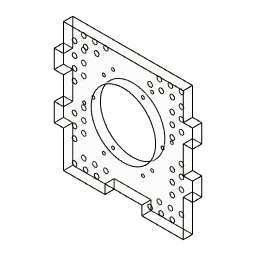
front_and_back_plates (Autodesk Fusion 360 design; units mm, degrees)
Autodesk Fusion 360 part; units mm, degrees
note: some values were not read from the file. Set by a fixed rule: which sketch regions a step uses.
sketch "Esquisse1" plane through (0, 0, 0) normal (0, 1, 0) x (1, 0, 0)
  line L0 (75, 75) -> (-75, 75) construction
  line L1 (-75, 75) -> (-75, -75) construction
  line L2 (-75, -75) -> (75, -75) construction
  line L3 (75, -75) -> (75, 75) construction
  line L4 (75, 75) -> (-75, -75) construction
  line L5 (-75, 75) -> (75, -75) construction
  circle A0 centre (0, 0) radius 35
  circle A1 centre (0, 0) radius 42.5 construction
  circle A2 centre (42.5, 0) radius 1.6
  line L6 (42.5, 0) -> (21.25, 36.8061) construction
  line L7 (21.25, 36.8061) -> (-21.25, 36.8061) construction
  line L8 (-21.25, 36.8061) -> (-42.5, 0) construction
  line L9 (-42.5, 0) -> (-21.25, -36.8061) construction
  line L10 (-21.25, -36.8061) -> (21.25, -36.8061) construction
  line L11 (21.25, -36.8061) -> (42.5, 0) construction
  circle A3 centre (21.25, -36.8061) radius 1.6
  circle A4 centre (-21.25, -36.8061) radius 1.6
  circle A5 centre (-42.5, 0) radius 1.6
  circle A6 centre (-21.25, 36.8061) radius 1.6
  circle A7 centre (21.25, 36.8061) radius 1.6
  line L12 (-65, -65) -> (0, -65)
  line L13 (0, -75) -> (0, 75)
  line L14 (-75, 0) -> (75, 0)
  line L15 (65, -65) -> (0, -65)
  line L16 (-65, 65) -> (0, 65) construction
  line L17 (65, 65) -> (0, 65) construction
  line L18 (-65, 35) -> (-65, 65)
  line L19 (-65, 35) -> (-75, 35)
  line L20 (-75, -75) -> (-75, 75) construction
  line L21 (-75, 15) -> (-65, 15)
  line L22 (-65, 15) -> (-65, 0.2731)
  line L23 (75, 75) -> (75, -75) construction
  line L24 (-75, 15) -> (-75, 35)
  line L25 (-65, -65) -> (-65, -35)
  line L26 (-65, -35) -> (-75, -35)
  line L27 (-75, -15) -> (-65, -15)
  line L28 (-65, -15) -> (-65, 0.2731)
  line L29 (-65, -65) -> (-65, 75) construction
  line L30 (-75, -15) -> (-75, -35)
  line L31 (65, -15) -> (65, 0.2731)
  line L32 (65, -65) -> (65, -35)
  line L33 (75, 15) -> (75, 35)
  line L34 (65, 35) -> (75, 35)
  line L35 (75, -15) -> (75, -35)
  line L36 (75, 15) -> (65, 15)
  line L37 (65, 15) -> (65, 0.2731)
  line L38 (65, -35) -> (75, -35)
  line L39 (65, 35) -> (65, 65)
  line L40 (75, -15) -> (65, -15)
  line L41 (-65, 65) -> (-65, 75)
  line L42 (-65, 75) -> (-20, 75)
  line L43 (-20, 75) -> (-20, 65)
  line L44 (-20, 65) -> (20, 65)
  line L45 (20, 65) -> (20, 75)
  line L46 (20, 75) -> (65, 75)
  line L47 (65, 75) -> (65, 65)
  circle A8 centre (0, 0) radius 50 construction
  point P0 (75, 0)
  point P1 (-75, -25)
  point P2 (-75, 25)
  dimension "d1" = 150
  dimension "d2" = 150
  dimension "d3" = 70
  dimension "d4" = 7.5
  dimension "d5" = 3.2
  dimension "d9" = 10
  dimension "d22" = 20
  dimension "d24" = 20
  dimension "d25" = 10
  dimension "d32" = 40
  dimension "d56" = 15
  dimension "d58" = 50
  constraint horizontal L0
  constraint perpendicular L0 L1
  constraint parallel L1 L3
  constraint coincident L4 A0.centre
  constraint coincident L5 A0.centre
  constraint coincident A0.centre A1.centre
  constraint concentric A0 A1
  constraint coincident A1 A2.centre
  constraint coincident A2.centre L6.start
  constraint coincident L10.end L11.start
  constraint coincident L9.end L10.start
  constraint coincident L8.end L9.start
  constraint coincident L7.end L8.start
  constraint coincident L6.end L7.start
  constraint equal A3 A4
  constraint equal A4 A5
  constraint equal A5 A6
  constraint equal A6 A7
  constraint equal A2 A7
  constraint perpendicular L1 L12
  constraint midpoint L2 L13.start
  constraint midpoint L0 L13.end
  constraint midpoint L1 L14.start
  constraint midpoint L3 P0
  constraint symmetric L12.start L13 L15.start
  constraint symmetric L12.end L13 L15.end
  constraint symmetric L0.start L14 L2.end
  constraint symmetric L0.end L14 L1.end
  constraint symmetric L1.end L14 L0.end
  constraint symmetric L2.end L14 L0.start
  constraint symmetric L12.start L14 L16.start
  constraint symmetric L12.end L14 L16.end
  constraint symmetric L14 L15.start L17.start
  constraint symmetric L14 L12.end L16.end
  constraint coincident A2.centre L14
  constraint perpendicular L12 L25
  constraint coincident L1 L26.end
  constraint perpendicular L1 L26
  constraint coincident L1 L27.start
  constraint perpendicular L1 L27
  constraint perpendicular L14 L28
  constraint coincident L0 L29.end
  constraint perpendicular L0 L29
  constraint coincident L12.start L28
  constraint vertical L24
  constraint coincident L1 L21.start
  constraint symmetric L13 L14.start P0
  constraint symmetric L13 L16.start L17.start
  constraint symmetric L13 L18.start L34.start
  constraint symmetric L13 L19.end L33.end
  constraint symmetric L13 L21.start L33.start
  constraint symmetric L13 L21.end L36.end
  constraint symmetric L13 L22.end L31.end
  constraint symmetric L13 L25.end L32.end
  constraint symmetric L13 L26.end L35.end
  constraint symmetric L13 L27.start L35.start
  constraint symmetric L13 L27.end L31.start
  constraint vertical L22
  constraint coincident L0 L42.end
  constraint coincident L16 L43.end
  constraint perpendicular L16 L43
  constraint coincident L17 L44.end
  constraint perpendicular L43 L44
  constraint coincident L0 L45.end
  constraint perpendicular L0 L45
  constraint coincident L0 L46.end
  constraint perpendicular L17 L47
  constraint symmetric L13 L43.end L44.end
  constraint vertical L18
  constraint concentric A1 A8
  constraint symmetric L14 L21.end L27.end
  constraint midpoint L30 P1
  constraint midpoint L24 P2
  measures "d1" distance of L1.end L2.end
  measures "d2" distance of L0.end L1.end
  measures "d3" diameter of A0
  measures "d4" distance of A0 A1
  measures "d5" diameter of A3
  measures "d9" distance of L2 L12
  measures "d22" distance of L19 L21
  measures "d24" distance of L26 L27
  measures "d25" distance of L20 L29
  measures "d32" distance of L43 L45
  measures "d56" distance of A0 A8
  measures "d58" distance of P1 P2
extrude "Extrusion1" add sketch "Esquisse1" along normal blind 10 contours A0 A2 L13 L14 L15 L31 L32 L35 L38 L40 | A0 A2 L13 L14 L31 L33 L34 L36 L37 L39 L44 L45 L46 L47 | A0 A5 L13 L14 L18 L19 L21 L22 L24 L28 L41 L42 L43 L44 | A0 A5 L12 L13 L14 L25 L26 L27 L28 L30
sketch "Esquisse3" plane through (0, 0, 0) normal (0, -1, 0) x (1, 0, 0)
  line L0 (65, 65) -> (-65, 65)
  line L1 (-65, 65) -> (-65, 35)
  line L2 (-65, 35) -> (-75, 35)
  line L3 (-75, 35) -> (-75, 15)
  line L4 (-75, 15) -> (-65, 15)
  line L5 (-65, 15) -> (-65, -15)
  line L6 (-65, -15) -> (-75, -15)
  line L7 (-75, -15) -> (-75, -35)
  line L8 (-75, -35) -> (-65, -35)
  line L9 (-65, -35) -> (-65, -75)
  line L10 (-65, -75) -> (-20, -75)
  line L11 (-20, -75) -> (-20, -65)
  line L12 (-20, -65) -> (20, -65)
  line L13 (20, -65) -> (20, -75)
  line L14 (20, -75) -> (65, -75)
  line L15 (65, -75) -> (65, -35)
  line L16 (65, -35) -> (75, -35)
  line L17 (75, -35) -> (75, -15)
  line L18 (75, -15) -> (65, -15)
  line L19 (65, -15) -> (65, 15)
  line L20 (65, 15) -> (75, 15)
  line L21 (75, 15) -> (75, 35)
  line L22 (75, 35) -> (65, 35)
  line L23 (65, 35) -> (65, 65)
  circle A0 centre (-42.5, 0) radius 1.6
  circle A1 centre (21.25, 36.8061) radius 1.6
  circle A2 centre (21.25, -36.8061) radius 1.6
  circle A3 centre (-21.25, -36.8061) radius 1.6
  circle A4 centre (42.5, 0) radius 1.6
  circle A5 centre (-21.25, 36.8061) radius 1.6
  circle A6 centre (0, 0) radius 35
  line L24 (-65, -64.8) -> (65, -64.8) construction
  line L25 (-65, -62.3) -> (65, -62.3) construction
  circle A7 centre (-53, -62.3) radius 2.5
  circle A8 centre (-41, -62.3) radius 2.5
  circle A9 centre (-29, -62.3) radius 2.5
  line L26 (0, -64.8) -> (0, 65)
  circle A10 centre (41, -62.3) radius 2.5
  circle A11 centre (53, -62.3) radius 2.5
  circle A12 centre (29, -62.3) radius 2.5
  line L27 (-53, -75) -> (-53, 65) construction
  circle A13 centre (-53, -39) radius 2.5
  circle A14 centre (-53, -27) radius 2.5
  circle A15 centre (-53, -15) radius 2.5
  circle A16 centre (-53, 15) radius 2.5
  circle A17 centre (-53, 27) radius 2.5
  circle A18 centre (-53, 39) radius 2.5
  line L28 (-65, 0) -> (65, 0)
  circle A19 centre (53, -15) radius 2.5
  circle A20 centre (53, 39) radius 2.5
  circle A21 centre (53, -39) radius 2.5
  circle A22 centre (53, 15) radius 2.5
  circle A23 centre (53, 27) radius 2.5
  circle A24 centre (53, -27) radius 2.5
  line L29 (53, -75) -> (53, 65) construction
  line L30 (-53, 53) -> (53, 53) construction
  circle A25 centre (-53, 53) radius 2.5
  circle A26 centre (-41, 53) radius 2.5
  circle A27 centre (-29, 53) radius 2.5
  line L31 (-41, 53) -> (-41, -62.3) construction
  line L32 (-29, 53) -> (-29, -62.3) construction
  circle A28 centre (53, 53) radius 2.5
  circle A29 centre (29, 53) radius 2.5
  circle A30 centre (41, 53) radius 2.5
  circle A31 centre (0, 0) radius 50 construction
  point P0 (41, 53)
  point P1 (53, 53)
  point P2 (29, 53)
  dimension "d33" = 0.2
  dimension "d34" = 5
  dimension "d36" = 12
  dimension "d37" = 12
  dimension "d38" = 12
  dimension "d39" = 5
  dimension "d40" = 5
  dimension "d41" = 5
  dimension "d42" = 5
  dimension "d43" = 5
  dimension "d44" = 5
  dimension "d45" = 12
  dimension "d46" = 12
  dimension "d47" = 12
  dimension "d48" = 12
  dimension "d49" = 30
  dimension "d50" = 12
  dimension "d51" = 5
  dimension "d52" = 5
  dimension "d53" = 5
  dimension "d54" = 12
  dimension "d57" = 15
  constraint coincident L9 L24.start
  constraint coincident L15 L24.end
  constraint perpendicular L15 L24
  constraint coincident L9 L25.start
  constraint coincident L15 L25.end
  constraint perpendicular L15 L25
  constraint coincident L25 A7.centre
  constraint coincident L25 A8.centre
  constraint coincident L25 A9.centre
  constraint equal A8 A9
  constraint equal A7 A8
  constraint tangent L24 A7
  constraint midpoint L24 L26.start
  constraint midpoint L0 L26.end
  constraint symmetric A7 L26 A11
  constraint symmetric A8 L26 A10
  constraint symmetric A9 L26 A12
  constraint coincident L10 L27.start
  constraint coincident L0 L27.end
  constraint perpendicular L0 L27
  constraint coincident L27 A13.centre
  constraint coincident L27 A14.centre
  constraint coincident L27 A15.centre
  constraint coincident L27 A16.centre
  constraint coincident L27 A17.centre
  constraint coincident L27 A18.centre
  constraint midpoint L5 L28.start
  constraint midpoint L19 L28.end
  constraint symmetric A15.centre A16.centre L28
  constraint symmetric L26 L27.start L29.start
  constraint symmetric L26 L27.end L29.end
  constraint symmetric L26 A13 A21
  constraint symmetric L26 A14 A24
  constraint symmetric L26 A15 A19
  constraint symmetric L26 A16 A22
  constraint symmetric L26 A17 A23
  constraint symmetric L26 A18 A20
  constraint coincident L27 L30.start
  constraint coincident L29 P1
  constraint perpendicular L29 L30
  constraint coincident L30.start A25.centre
  constraint coincident L30 A26.centre
  constraint coincident L30 A27.centre
  constraint coincident A26.centre L31.start
  constraint coincident A8.centre L31.end
  constraint coincident A27.centre L32.start
  constraint coincident A9.centre L32.end
  constraint vertical L32
  constraint vertical L31
  constraint symmetric L26 L30.start P1
  constraint symmetric L26 A25 A28
  constraint symmetric L26 A26 A30
  constraint symmetric L26 A27 A29
  constraint symmetric L26 A26.centre P0
  constraint symmetric L26 A27.centre P2
  constraint coincident A6.centre A31.centre
  measures "d33" distance of L12 L24
  measures "d34" diameter of A7
  measures "d36" distance of A7.centre A8.centre
  measures "d37" distance of A8.centre A9.centre
  measures "d38" distance of L25.start A7.centre
  measures "d39" diameter of A13
  measures "d40" diameter of A14
  measures "d41" diameter of A15
  measures "d42" diameter of A16
  measures "d43" diameter of A17
  measures "d44" diameter of A18
  measures "d45" distance of A13.centre A14.centre
  measures "d46" distance of A14.centre A15.centre
  measures "d47" distance of A16.centre A17.centre
  measures "d48" distance of A17.centre A18.centre
  measures "d49" distance of A15.centre A16.centre
  measures "d50" distance of L1 L27
  measures "d51" diameter of A25
  measures "d52" diameter of A26
  measures "d53" diameter of A27
  measures "d54" distance of L0 L30
  measures "d57" distance of A6 A31
extrude "Extrusion3" cut sketch "Esquisse3" against normal through all contours A7 | A8 | A9 | A10 | A11 | A12 | A13 | A14 | A15 | A16 | A17 | A18 | A19 | A20 | A21 | A22 | A23 | A24 | A25 | A26 | A27 | A28 | A29 | A30
